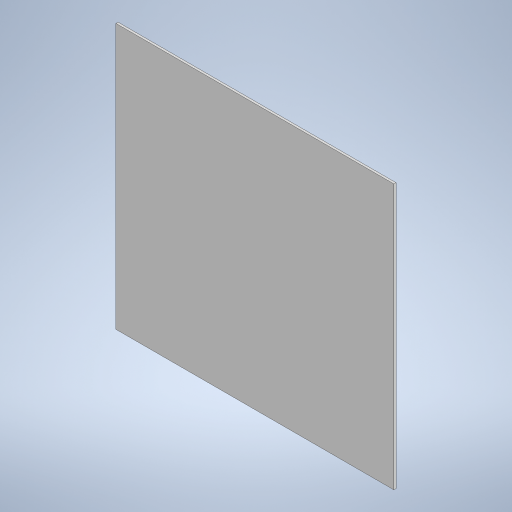
# Autodesk Inventor part: big_back_plywood_Ocampo
Saved by Autodesk Inventor 2023 (Build 270158000, 158)
## iProperties
Created: 2025-02-24
Part Number: big_back_plywood_Ocampo
Material: Generic
Document SubType Name: Modeling
Designer: 1244275
Density: 1 g/cm^3
Appearance: Default
Author: 1244275
Autodesk Inventor part; units mm, degrees
ref_plane "YZ Plane" through (0, 0, 0) normal (1, 0, 0) x (0, 1, 0)
ref_plane "XZ Plane" through (0, 0, 0) normal (0, 1, 0) x (-1, 0, 0)
ref_plane "XY Plane" through (0, 0, 0) normal (0, 0, 1) x (1, 0, 0)
sketch "Sketch1" plane through (0, 0, 0) normal (0, 0, 1) x (1, 0, 0)
  line L0 (0, 0) -> (812.8, 0)
  line L1 (812.8, 0) -> (812.8, 762)
  line L2 (812.8, 762) -> (0, 762)
  line L3 (0, 762) -> (0, 0)
  dimension "d0" = 812.8
  dimension "d1" = 762
  constraints: 8 end point, 2 parallel, 1 horizontal, 1 perpendicular
  measures "d0" distance of L2.end L1.end
  measures "d1" distance of L1.end L0.end
extrude "Extrusion1" add sketch "Sketch1" along normal blind 6.35
sketch "Sketch2" plane through (0, 0, 0) normal (0, 0, 1) x (1, 0, 0)
  line L0 (0, 762) -> (0, 0) projected
  line L1 (0, 0) -> (0, -12.7)
  line L2 (0, -12.7) -> (812.8, -12.7)
  line L3 (0, 0) -> (812.8, 0) projected
  line L4 (812.8, -12.7) -> (812.8, 0)
  line L5 (812.8, 0) -> (0, 0)
  dimension "d4" = 12.7
  constraints: 8 end point, 2 equal length, 1 perpendicular, 1 vertical
  measures "d4" distance of L0.end L1.end
extrude "Extrusion2" add sketch "Sketch2" along normal blind 6.35
body "Solid1"
